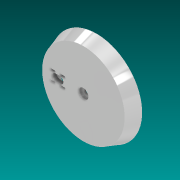
# Autodesk Inventor part: base bovenkant v2
Saved by Autodesk Inventor 2020.2 (Build 242310000, 310)
## iProperties
Created: 2020-05-15
Part Number: base bovenkant v2
Material: Aluminum 6061
Document SubType Name: Modeling
Designer: Svend
Density: 2.7 g/cm^3
Appearance: Aluminum - Polished
Author: Svend
Autodesk Inventor part; units mm, degrees
ref_plane "YZ Plane" through (0, 0, 0) normal (1, 0, 0) x (0, 1, 0)
ref_plane "XZ Plane" through (0, 0, 0) normal (0, 1, 0) x (-1, 0, 0)
ref_plane "XY Plane" through (0, 0, 0) normal (0, 0, 1) x (1, 0, 0)
sketch "Sketch1" plane through (0, 0, 0) normal (0, 0, 1) x (1, 0, 0)
  circle A0 centre (-11.3135, -11.3135) radius 2
  circle A1 centre (-11.3135, 11.3135) radius 2
  circle A2 centre (11.3135, 11.3135) radius 2
  circle A3 centre (11.3135, -11.3135) radius 2
  circle A4 centre (-15.3135, 11.3135) radius 2
  circle A5 centre (-7.3135, 11.3135) radius 2
  circle A6 centre (7.3135, 11.3135) radius 2
  circle A7 centre (15.3135, 11.3135) radius 2
  circle A8 centre (15.3135, -11.3135) radius 2
  circle A9 centre (7.3135, -11.3135) radius 2
  circle A10 centre (-7.3135, -11.3135) radius 2
  circle A11 centre (-15.3135, -11.3135) radius 2
  line L0 (-15.3135, 13.3135) -> (-7.3135, 13.3135)
  line L1 (-7.3135, 9.3135) -> (-15.3135, 9.3135)
  line L2 (-15.3135, -9.3135) -> (-7.3135, -9.3135)
  line L3 (-7.3135, -13.3135) -> (-15.3135, -13.3135)
  line L4 (7.3135, -9.3135) -> (15.3135, -9.3135)
  line L5 (15.3135, -13.3135) -> (7.3135, -13.3135)
  line L6 (15.3135, 9.3135) -> (7.3135, 9.3135)
  line L7 (15.3135, 13.3135) -> (7.3135, 13.3135)
  circle A12 centre (0, 0) radius 8.25
  circle A13 centre (5, 0) radius 8.25
  circle A14 centre (-5, 0) radius 8.25
  line L8 (-5, 8.25) -> (5, 8.25)
  line L9 (5, -8.25) -> (-5, -8.25)
  circle A15 centre (0, 0) radius 42.5
  circle A16 centre (59.509, 0) radius 50.7821
  line L10 (-5.9149, 42.0864) -> (52.4415, 50.2878)
  line L11 (-5.9149, -42.0864) -> (52.4415, -50.2878)
  line L12 (-13.25, 0) -> (13.25, 0)
  circle A17 centre (59.509, 0) radius 11.5
  arc A18 (-5.9149, 42.0864) -> (-5.9149, -42.0864) centre (0, 0) ccw
  line L13 (-42.5, 0) -> (156.5802, 0)
  circle A19 centre (59.509, 0) radius 85
  point P0 (-3.1314, -32.3793)
  point P1 (23.2633, -35.5678)
  point P2 (23.2633, 35.5678)
  dimension "d0" = 4
  dimension "d1" = 22.627
  dimension "d2" = 22.627
  dimension "d3" = 11.3135
  dimension "d4" = 11.3135
  dimension "d5" = 4
  dimension "d6" = 4
  dimension "d7" = 4
  dimension "d8" = 4
  dimension "d9" = 4
  dimension "d10" = 4
  dimension "d11" = 4
  dimension "d12" = 4
  dimension "d15" = 16.5
  dimension "d16" = 5
  dimension "d17" = 5
  dimension "d18" = 85
  dimension "d19" = 8
  dimension "d20" = 59.509
  dimension "d21" = 23
  dimension "d24" = 85
  dimension "d116" = 170
  constraints: 29 point on circle, 28 end point, 20 centre point, 13 equal radius, 13 horizontal alignment, 10 tangent, 9 point on line, 5 coincident, 4 parallel, 3 horizontal, 2 midpoint, 2 vertical alignment
  measures "d0" diameter of A0
  measures "d1" distance of A1.centre A2.centre
  measures "d2" distance of A3.centre A2.centre
  measures "d3" horizontal distance of point (0, 0) A1.centre
  measures "d4" horizontal distance of point (0, 0) A1.centre
  measures "d5" distance of A2.centre A6.centre
  measures "d6" distance of A7.centre A2.centre
  measures "d7" distance of A3.centre A8.centre
  measures "d8" distance of A9.centre A3.centre
  measures "d9" distance of A0.centre A10.centre
  measures "d10" distance of A11.centre A0.centre
  measures "d11" distance of A1.centre A4.centre
  measures "d12" distance of A5.centre A1.centre
  measures "d15" diameter of A12
  measures "d16" distance of A14.centre A12.centre
  measures "d17" distance of A12.centre A13.centre
  measures "d18" diameter of A15
  measures "d19" angle of L12 L10
  measures "d20" distance of A16.centre point (0, 0)
  measures "d21" diameter of A17
  measures "d24" diameter of A18
  measures "d116" diameter of A19
extrude "Extrusion1" add sketch "Sketch1" along normal blind 10 contours L7 A16 A15 L13 A13 L6 A7 | L7 A6 L6 A16 A13 L8 A14 L13 A19 A15 | A16 L13 A17 A15 | A15 L10 A16 | L13 A17 A16 A15 | A15 A16 L5 A8 L4 A13 L13 | A15 A19 L13 A16 L10 | A16 L11 A15 | A15 A19 L13 A14 L9 A13 A16 L4 A9 L5 | L13 A19 A15 L11 A16
sketch "Sketch15" plane through (0, 0, 0) normal (0, 1, 0) x (-1, 0, 0)
  line L0 (25.491, 10) -> (-144.509, 10) projected
  line L1 (-71.009, 10) -> (-48.009, 10) projected
  line L2 (-15.3135, 10) -> (-7.3135, 10) projected
  line L3 (-7.3135, 10) -> (-7.3135, 10) projected
  line L4 (-7.3135, 10) -> (-15.3135, 10) projected
  line L5 (-15.3135, 10) -> (-15.3135, 10) projected
  line L6 (7.3135, 10) -> (15.3135, 10) projected
  line L7 (15.3135, 10) -> (15.3135, 10) projected
  line L8 (15.3135, 10) -> (7.3135, 10) projected
  line L9 (7.3135, 10) -> (7.3135, 10) projected
  line L10 (-15.3135, 10) -> (-7.3135, 10) projected
  line L11 (-7.3135, 10) -> (-7.3135, 10) projected
  line L12 (-7.3135, 10) -> (-15.3135, 10) projected
  line L13 (-15.3135, 10) -> (-15.3135, 10) projected
  line L14 (7.3135, 10) -> (15.3135, 10) projected
  line L15 (15.3135, 10) -> (15.3135, 10) projected
  line L16 (15.3135, 10) -> (7.3135, 10) projected
  line L17 (7.3135, 10) -> (7.3135, 10) projected
  line L18 (5, 10) -> (5, 10) projected
  line L19 (5, 10) -> (-5, 10) projected
  line L20 (-5, 10) -> (-5, 10) projected
  line L21 (-5, 10) -> (5, 10) projected
  line L22 (-71.009, 10) -> (-71.009, 0) projected
  line L23 (-48.009, 10) -> (-48.009, 0) projected
  line L24 (-15.3135, 0) -> (-15.3135, 10) projected
  line L25 (-13.25, 10) -> (-13.25, 0) projected
  line L26 (13.25, 10) -> (13.25, 0) projected
  line L27 (25.491, 0) -> (25.491, 10) projected
  line L28 (25.491, 0) -> (-144.509, 0) projected
  line L29 (-71.009, 0) -> (-48.009, 0) projected
  line L30 (-15.3135, 0) -> (-7.3135, 0) projected
  line L31 (-15.3135, 0) -> (-15.3135, 0) projected
  line L32 (-7.3135, 0) -> (-15.3135, 0) projected
  line L33 (-7.3135, 0) -> (-7.3135, 0) projected
  line L34 (7.3135, 0) -> (15.3135, 0) projected
  line L35 (7.3135, 0) -> (7.3135, 0) projected
  line L36 (15.3135, 0) -> (7.3135, 0) projected
  line L37 (15.3135, 0) -> (15.3135, 0) projected
  line L38 (-15.3135, 0) -> (-7.3135, 0) projected
  line L39 (-15.3135, 0) -> (-15.3135, 0) projected
  line L40 (-7.3135, 0) -> (-15.3135, 0) projected
  line L41 (-7.3135, 0) -> (-7.3135, 0) projected
  line L42 (7.3135, 0) -> (15.3135, 0) projected
  line L43 (7.3135, 0) -> (7.3135, 0) projected
  line L44 (15.3135, 0) -> (7.3135, 0) projected
  line L45 (15.3135, 0) -> (15.3135, 0) projected
  line L46 (5, 0) -> (5, 0) projected
  line L47 (-5, 0) -> (5, 0) projected
  line L48 (-5, 0) -> (-5, 0) projected
  line L49 (5, 0) -> (-5, 0) projected
  line L50 (25.491, 10) -> (35.491, 10)
  line L51 (35.491, 10) -> (35.491, -20)
  line L52 (35.491, -20) -> (25.491, -20)
  line L53 (25.491, -20) -> (25.491, 10)
  line L54 (-59.509, 10) -> (-59.509, 0)
  line L55 (35.491, 10) -> (45.491, -20)
  line L56 (45.491, -20) -> (35.491, -20)
  circle A0 centre (35.491, -21) radius 7.5
  point P0 (0, 0)
  point P1 (28.058, -20)
  point P2 (42.924, -20)
  dimension "d117" = 10
  dimension "d118" = 30
  dimension "d120" = 10
  dimension "d122" = 15
  dimension "d123" = 1
  constraints: 14 end point, 2 horizontal, 2 midpoint, 2 parallel, 1 centre point, 1 perpendicular, 1 vertical alignment
  measures "d117" distance of L51.end L52.end
  measures "d118" distance of L50.end L51.end
  measures "d120" distance of L55.end L51.end
  measures "d122" diameter of A0
  measures "d123" distance from line of L52 A0.centre
revolve "Revolution4" add sketch "Sketch15" angle 360 about axis through (59.509, 0, 10) along (0, 0, -1) contours L50 L51 A0 L52 L53 L27 | L55 L56 A0 L51
sketch "Sketch16" plane through (59.509, 0, 0) normal (0, 0, -1) x (-1, 0, 0)
  circle A0 centre (0, 0) radius 11.5 projected
  circle A1 centre (0, 0) radius 4.5
  point P0 (59.509, 0)
  dimension "d124" = 9
  constraints: 1 centre point, 1 coincident
  measures "d124" diameter of A1
extrude "Extrusion8" add sketch "Sketch16" against normal blind 3
equation "\"d2\" = d1"
equation "\"d3\" = 0.5 * d2"
equation "\"d4\" = 0.5 * d1"
equation "\"d5\" = d0"
equation "\"d6\" = d5"
equation "\"d7\" = d6"
equation "\"d8\" = d7"
equation "\"d9\" = d5"
equation "\"d10\" = d9"
equation "\"d11\" = d10"
equation "\"d12\" = d11"
equation "\"d17\" = d16"
body "Solid1"
